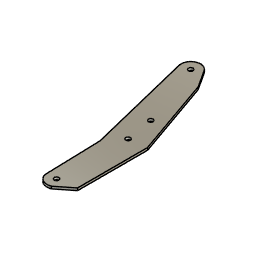
LIGHTS_SIDE_PLATE (Autodesk Fusion 360 design; units mm, degrees)
Autodesk Fusion 360 part; units mm, degrees
sketch "Esquisse1" plane through (0, 0, 0) normal (0, 0, 1) x (1, 0, 0)
  circle A0 centre (-28.9762, 57.1678) radius 4 construction
  circle A1 centre (0, 0) radius 4 construction
  circle A2 centre (65.0769, 11.2557) radius 4 construction
  spline S0 degree 3 poles (-28.9762, 70.1678) (-36.1559, 70.1678) (-41.9762, 64.3475) (-41.9762, 57.1678) (-41.9762, 49.9881) (-36.1559, 44.1678) (-28.9762, 44.1678) knots 0 0 0 0 1 1 1 2 2 2 2
  spline S1 degree 3 poles (-10.2665, 7.9748) (-2.9429, 18.3079) (-5.3826, 32.6214) (-15.7156, 39.945) (-19.5917, 42.6922) (-24.2253, 44.1678) (-28.9762, 44.1678) knots 0 0 0 0 1 1 1 2 2 2 2
  spline S2 degree 3 poles (64.1314, 172.9751) (62.374, 174.7324) (59.5248, 174.7324) (57.7674, 172.9751) (56.0101, 171.2177) (56.0101, 168.3685) (57.7674, 166.6111) knots 0 0 0 0 1 1 1 2 2 2 2
  line L0 (70.1314, 166.9751) -> (64.1314, 172.9751) construction
  spline S3 degree 3 poles (63.7674, 160.6111) (65.5248, 158.8538) (68.374, 158.8538) (70.1314, 160.6111) (71.8888, 162.3685) (71.8888, 165.2177) (70.1314, 166.9751) knots 0 0 0 0 1 1 1 2 2 2 2
  line L1 (63.7674, 160.6111) -> (57.7674, 166.6111) construction
  spline S4 degree 3 poles (48.9494, 163.7931) (48.9494, 162.9431) (49.0096, 162.0942) (49.1296, 161.2528) knots 0 0 0 0 1 1 1 1
  line L2 (57.7674, 166.6111) -> (63.7674, 160.6111) construction
  spline S5 degree 3 poles (64.1314, 172.9751) (62.374, 174.7324) (59.5248, 174.7324) (57.7674, 172.9751) (56.0101, 171.2177) (56.0101, 168.3685) (57.7674, 166.6111) knots 0 0 0 0 1 1 1 2 2 2 2 construction
  line L3 (70.1314, 166.9751) -> (64.1314, 172.9751) construction
  spline S6 degree 3 poles (63.7674, 160.6111) (65.5248, 158.8538) (68.374, 158.8538) (70.1314, 160.6111) (71.8888, 162.3685) (71.8888, 165.2177) (70.1314, 166.9751) knots 0 0 0 0 1 1 1 2 2 2 2 construction
  circle A3 centre (77.1957, 405.5301) radius 9.525 construction
  spline S7 degree 3 poles (-10.2665, 7.9748) (-2.9429, 18.3079) (-5.3826, 32.6214) (-15.7156, 39.945) (-19.5917, 42.6922) (-24.2253, 44.1678) (-28.9762, 44.1678) knots 0 0 0 0 1 1 1 2 2 2 2 construction
  spline S8 degree 3 poles (-10.2665, 7.9748) (-14.6709, 2.3048) (-13.6449, -5.8622) (-7.9748, -10.2665) (-5.0869, -12.5098) (-1.3877, -13.433) (2.2156, -12.8098) knots 0 0 0 0 1 1 1 2 2 2 2 construction
  circle A4 centre (66.9494, 163.7931) radius 4.5 construction
  circle A5 centre (66.9494, 163.7931) radius 2.95 construction
  circle A6 centre (77.1957, 405.5301) radius 6.2 construction
  arc A7 (29.3943, 70.1678) -> (38.5415, 76.1229) centre (29.3943, 80.1706) ccw construction
  circle A8 centre (105.659, 34.9839) radius 3 construction
  line L4 (30.2663, 244.3325) -> (62.716, 371.2499) construction
  line L5 (150.2746, 456.2058) -> (249.6046, 17.5293) construction
  line L6 (66.9494, 163.7931) -> (35.3654, 116.3437) construction
  circle A9 centre (86.9154, 445.0854) radius 2 construction
  line L7 (86.9154, 445.0854) -> (59.0066, 452.9658) construction
  line L8 (59.0066, 452.9658) -> (50.8545, 424.0946) construction
  line L9 (59.0066, 452.9658) -> (67.1587, 481.8369) construction
  circle A10 centre (-28.9762, 57.1678) radius 13.0029 construction
  circle A11 centre (0, 0) radius 13.0029 construction
  circle A12 centre (105.659, 34.9839) radius 13 construction
  circle A13 centre (146.3497, 66.662) radius 3 construction
  circle A14 centre (146.3497, 66.662) radius 7.5 construction
  circle A15 centre (66.9494, 163.7931) radius 13 construction
  line L10 (30.2663, 244.3325) -> (49.643, 239.3784) construction
  line L11 (49.643, 239.3784) -> (82.0927, 366.2958) construction
  line L12 (194.3502, 181.1189) -> (109.3502, 181.1189) construction
  line L13 (109.3502, 181.1189) -> (109.3502, 117.1189) construction
  line L14 (109.3502, 117.1189) -> (194.3502, 117.1189) construction
  line L15 (194.3502, 117.1189) -> (194.3502, 181.1189) construction
  line L16 (89.3502, 252.2924) -> (174.3502, 252.2924) construction
  line L17 (174.3502, 252.2924) -> (174.3502, 188.2924) construction
  line L18 (174.3502, 188.2924) -> (89.3502, 188.2924) construction
  line L19 (89.3502, 188.2924) -> (89.3502, 252.2924) construction
  arc A16 (149.7785, 59.9917) -> (116.6647, 28.0647) centre (186.2634, -10.9854) ccw construction
  arc A17 (-10.2665, 7.9748) -> (6.9982, -10.9556) centre (0, 0) ccw construction
  line L20 (115, 102) -> (155, 102) construction
  line L21 (155, 102) -> (155, 82) construction
  line L22 (155, 82) -> (115, 82) construction
  line L23 (115, 82) -> (115, 102) construction
  spline S9 degree 5 poles (47.7274, 67.4718) (47.3281, 66.25) (46.4427, 63.9241) (44.8543, 60.7877) (42.2069, 57.3229) (37.9663, 54.2531) (32.7422, 52.5151) (26.5189, 52.1302) (19.36, 53.0121) (11.3588, 55.0347) (2.6106, 58.0689) (-4.924, 61.2221) (-10.8549, 63.966) (-14.9312, 65.9611) (-17, 67) knots 0 0 0 0 0 0 0.1 0.2 0.3 0.4 0.5 0.6 0.7 0.8 0.9 1 1 1 1 1 1 construction
  arc A18 (149.7785, 59.9917) -> (145.7758, 74.1401) centre (146.3497, 66.662) ccw construction
  arc A19 (106.8583, 22.0393) -> (116.6647, 28.0647) centre (105.659, 34.9839) ccw construction
  line L24 (82.0927, 366.2958) -> (42.6573, 212.0556) construction
  spline S10 degree 5 poles (-17, 67) (-17.1898, 67.1027) (-17.5737, 67.3046) (-18.1631, 67.5968) (-18.9761, 67.9649) (-20.0408, 68.3868) (-21.1577, 68.7673) (-22.3305, 69.1037) (-23.5599, 69.3954) (-24.8424, 69.645) (-26.1736, 69.8562) (-27.2741, 69.9971) (-28.118, 70.0881) (-28.6888, 70.1423) (-28.9762, 70.1678) knots 0 0 0 0 0 0 0.1 0.2 0.3 0.4 0.5 0.6 0.7 0.8 0.9 1 1 1 1 1 1 construction
  line L25 (112.0927, 366.2958) -> (82.0927, 366.2958) construction
  circle A20 centre (0, 0) radius 4.15 construction
  circle A21 centre (-28.9762, 57.1678) radius 4.15 construction
  arc A22 (47.7274, 67.4718) -> (42.6713, 210.5165) centre (-255.8881, 128.3519) ccw construction
  circle A23 centre (66.9494, 163.7931) radius 3 construction
  circle A24 centre (110.8323, 274.6584) radius 7.5 construction
  arc A25 (106.8583, 22.0393) -> (6.9982, -10.9556) centre (128.4398, -210.8903) ccw construction
  arc A26 (82.0927, 366.2958) -> (71.4434, 397.9383) centre (52.352, 373.8997) ccw construction
  arc A27 (6.7295, -63.1083) -> (50.332, 237.2291) centre (-255.8881, 128.3519) ccw construction
  arc A28 (165.8909, 81.8045) -> (94.5564, -35.7811) centre (186.2634, -10.9854) ccw construction
  arc A29 (305.7966, -36.1174) -> (-67.5783, -57.3394) centre (128.4398, -210.8903) ccw construction
  line L26 (110.0008, 99.9968) -> (84.3502, 214.0814) construction
  arc A30 (112.5946, 267.3684) -> (84.3502, 214.0814) centre (122.0574, 228.2239) ccw construction
  arc A31 (110.0008, 99.9968) -> (145.7758, 74.1401) centre (143.1616, 108.2003) ccw construction
  line L27 (62.716, 371.2499) -> (30.2663, 244.3325) construction
  line L28 (30.2663, 244.3325) -> (-3.6429, 253.0023) construction
  line L29 (-3.6429, 253.0023) -> (28.8068, 379.9197) construction
  line L30 (28.8068, 379.9197) -> (62.716, 371.2499) construction
  line L31 (28.8068, 379.9197) -> (32.5224, 394.4522) construction
  line L32 (32.5224, 394.4522) -> (62.716, 371.2499) construction
  line L33 (-3.6429, 253.0023) -> (-7.3585, 238.4698) construction
  line L34 (-7.3585, 238.4698) -> (30.2663, 244.3325) construction
  arc A32 (112.0927, 366.2958) -> (115.0505, 280.8597) centre (180.406, 325.8915) ccw construction
  arc A33 (112.5946, 267.3684) -> (115.0505, 280.8597) centre (110.8323, 274.6584) ccw construction
  circle A34 centre (110.8323, 274.6584) radius 3 construction
  circle A35 centre (77.1957, 405.5301) radius 6 construction
  arc A36 (69.3852, 410.9818) -> (71.4434, 397.9383) centre (77.1957, 405.5301) ccw construction
  arc A37 (142.115, 85.3833) -> (84.2801, -39.8886) centre (186.2634, -10.9854) ccw construction
  arc A38 (108.2254, 142.5582) -> (166.09, 64.8957) centre (143.1616, 108.2003) ccw construction
  line L35 (69.7156, 210.791) -> (84.3502, 214.0814) construction
  line L36 (110.0008, 99.9968) -> (95.3661, 96.7063) construction
  line L37 (95.3661, 96.7063) -> (70.593, 206.8884) construction
  line L38 (65.813, 209.9136) -> (63.0859, 209.3004) construction
  line L39 (69.6598, 177.648) -> (72.9035, 178.3773) construction
  line L40 (71.751, 151.5603) -> (78.7024, 152.9702) construction
  line L41 (91.664, 95.874) -> (69.6275, 90.9193) construction
  line L42 (88.6169, 108.4898) -> (73.4183, 105.0726) construction
  line L43 (91.642, 113.2699) -> (83.4, 149.9274) construction
  line L44 (69.7156, 210.791) -> (75.9287, 183.1573) construction
  arc A39 (64.835, 180.9038) -> (60.0746, 204.4611) centre (-255.8881, 128.3519) ccw construction
  arc A40 (68.5478, 109.2108) -> (68.5529, 147.4056) centre (-255.8881, 128.3519) ccw construction
  arc A41 (58.4283, 45.7068) -> (66.5367, 87.5193) centre (-255.8881, 128.3519) ccw construction
  arc A42 (96.3504, 93.1926) -> (111.6523, 70.4686) centre (143.1616, 108.2003) ccw construction
  arc A43 (111.8948, 64.5481) -> (98.719, 48.7807) centre (186.2634, -10.9854) ccw construction
  arc A44 (95.9158, 47.0674) -> (63.299, 40.8172) centre (128.4398, -210.8903) ccw construction
  arc A45 (58.4283, 45.7068) -> (63.299, 40.8172) centre (62.2968, 44.6896) ccw construction
  arc A46 (69.6275, 90.9193) -> (66.5367, 87.5193) centre (70.505, 87.0168) ccw construction
  arc A47 (111.8948, 64.5481) -> (111.6523, 70.4686) centre (109.0884, 67.3984) ccw construction
  arc A48 (95.9158, 47.0674) -> (98.719, 48.7807) centre (95.4155, 51.036) ccw construction
  arc A49 (96.3504, 93.1926) -> (91.664, 95.874) centre (92.5414, 91.9714) ccw construction
  arc A50 (71.751, 151.5603) -> (68.5529, 147.4056) centre (72.546, 147.6401) ccw construction
  arc A51 (68.5478, 109.2108) -> (73.4183, 105.0726) centre (72.5408, 108.9752) ccw construction
  arc A52 (88.6169, 108.4898) -> (91.642, 113.2699) centre (87.7395, 112.3924) ccw construction
  arc A53 (83.4, 149.9274) -> (78.7024, 152.9702) centre (79.4974, 149.05) ccw construction
  arc A54 (72.9035, 178.3773) -> (75.9287, 183.1573) centre (72.0261, 182.2799) ccw construction
  arc A55 (64.835, 180.9038) -> (69.6598, 177.648) centre (68.7824, 181.5506) ccw construction
  arc A56 (63.0859, 209.3004) -> (60.0746, 204.4611) centre (63.9633, 205.3978) ccw construction
  arc A57 (70.593, 206.8884) -> (65.813, 209.9136) centre (66.6904, 206.011) ccw construction
  arc A58 (133.9714, 281.918) -> (103.7167, 176.372) centre (122.0574, 228.2239) ccw construction
  arc A59 (124.2253, 402.4992) -> (112.5946, 259.3587) centre (180.406, 325.8915) ccw construction
  line L45 (85.3019, 318.2923) -> (52.245, 189.4942) construction
  line L46 (78.1169, 264.0249) -> (74.6937, 264.9035) construction
  line L47 (72.533, 268.5524) -> (81.8866, 305.1363) construction
  arc A60 (87.72, 305.0513) -> (96.914, 280.5695) centre (180.406, 325.8915) ccw construction
  arc A61 (95.7143, 276.5047) -> (81.0969, 264.9286) centre (122.0574, 228.2239) ccw construction
  arc A62 (95.7143, 276.5047) -> (96.914, 280.5695) centre (94.2774, 279.1382) ccw construction
  arc A63 (87.72, 305.0513) -> (81.8866, 305.1363) centre (84.7931, 304.3932) ccw construction
  arc A64 (72.533, 268.5524) -> (74.6937, 264.9035) centre (75.4395, 267.8093) ccw construction
  arc A65 (78.1169, 264.0249) -> (81.0969, 264.9286) centre (78.8627, 266.9307) ccw construction
  arc A66 (42.6573, 212.0556) -> (42.6713, 210.5165) centre (45.5638, 211.3125) ccw construction
  circle A67 centre (86.9154, 445.0854) radius 7.5 construction
  arc A68 (94.3544, 446.0401) -> (112.0927, 366.2958) centre (365.6747, 464.5475) ccw construction
  arc A69 (69.3852, 410.9818) -> (79.4497, 445.8015) centre (7.9302, 447.6095) ccw construction
  arc A70 (94.3544, 446.0401) -> (79.4497, 445.8015) centre (86.9154, 445.0854) ccw construction
  line L48 (227.4805, 115.2371) -> (278.7067, 112.3358) construction
  line L49 (139.3502, 181.1189) -> (139.3502, 117.1189) construction
  line L50 (152.3502, 181.1189) -> (152.3502, 117.1189) construction
  line L51 (139.3502, 149.1189) -> (152.3502, 149.1189) construction
  line L52 (119.3502, 252.2924) -> (119.3502, 188.2924) construction
  line L53 (132.3502, 252.2924) -> (132.3502, 188.2924) construction
  line L54 (132.3502, 220.2924) -> (119.3502, 220.2924) construction
  circle A71 centre (110.8323, 274.6584) radius 3
  circle A72 centre (146.3497, 66.662) radius 3
  circle A73 centre (119.3502, 220.2924) radius 2.5 construction
  line L55 (155, 92) -> (147, 92) construction
  line L56 (98.4811, 272.7355) -> (132, 137)
  arc A74 (134.15, 63.9386) -> (151.2172, 55.1487) centre (146.3497, 66.662) ccw
  arc A75 (119.9733, 283.1844) -> (98.4811, 272.7355) centre (110.8323, 274.6584) ccw
  arc A76 (204.218, 109.7343) -> (203.7833, 111.288) centre (194.4019, 107.8255) ccw
  line L57 (134.15, 63.9386) -> (132, 137)
  line L58 (119.9733, 283.1844) -> (135, 260)
  line L59 (170, 70) -> (170, 160)
  line L60 (170, 160) -> (135, 260)
  line L61 (151.2172, 55.1487) -> (170, 70)
  circle A77 centre (149.3502, 129.1189) radius 2.5 construction
  circle A78 centre (141.8502, 192.2924) radius 3
  circle A79 centre (147.8502, 157.1189) radius 3
  point P0 (42.4595, 211.2822)
  point P1 (33.0466, 52.9627)
  point P2 (-22, 69)
  dimension "d3" = 5.9
  dimension "d4" = 12.4
  dimension "d49" = 6
  dimension "d53" = 131
  dimension "d64" = 4
  dimension "d68" = 29
  dimension "d69" = 30
  dimension "d70" = 30
  dimension "d71" = 26
  dimension "d72" = 6
  dimension "d73" = 15
  dimension "d74" = 26
  dimension "d75" = 20
  dimension "d76" = 30
  dimension "d77" = 160
  dimension "d78" = 64
  dimension "d79" = 85
  dimension "d80" = 64
  dimension "d81" = 85
  dimension "d82" = 20
  dimension "d83" = 40
  dimension "d86" = 8.3
  dimension "d87" = 8.3
  dimension "d88" = 6
  dimension "d89" = 15
  dimension "d93" = 79.8054
  dimension "d94" = 309.659
  dimension "d95" = 233.9273
  dimension "d97" = 325
  dimension "d98" = 95
  dimension "d99" = 249
  dimension "d104" = 35
  dimension "d105" = 15
  dimension "d106" = 15
  dimension "d107" = 6
  dimension "d108" = 12
  dimension "d109" = 106
  dimension "d111" = 49
  dimension "d112" = 15
  dimension "d113" = 4
  dimension "d114" = 4
  dimension "d115" = 4
  dimension "d116" = 4
  dimension "d117" = 4
  dimension "d118" = 55
  dimension "d119" = 95
  dimension "d121" = 3
  dimension "d122" = 3
  dimension "d123" = 3
  dimension "d124" = 3
  dimension "d131" = 3
  dimension "d132" = 15
  dimension "d133" = 74
  dimension "d135" = 55
  dimension "d137" = 42
  dimension "d138" = 42
  dimension "d139" = 13
  dimension "d141" = 5
  dimension "d142" = 8
  dimension "d153" = 35
  dimension "d154" = 55
  dimension "d156" = 5
  dimension "d157" = 10
  dimension "d158" = 20
  dimension "d164" = 6
  dimension "d165" = 22.5
  dimension "d166" = 28
  dimension "d170" = 6
  dimension "d171" = 1.5
  dimension "d172" = 28
  constraint coincident S3.start A4
  constraint coincident L0.start A4
  constraint tangent L3 A4
  constraint tangent L1 A4
  constraint concentric A4 A5
  constraint concentric A3 A6
  constraint coincident A4.centre A5.centre
  constraint coincident A9.centre L7.start
  constraint perpendicular L7 L8
  constraint perpendicular L7 L9
  constraint concentric A0 A10
  constraint concentric A8 A12
  constraint coincident A12 A19.start
  constraint concentric A13 A14
  constraint coincident A12 A16.end
  constraint concentric A4 A15
  constraint coincident L4.start L10.start
  constraint horizontal L12
  constraint vertical L13
  constraint horizontal L14
  constraint vertical L15
  constraint horizontal L16
  constraint vertical L17
  constraint horizontal L18
  constraint vertical L19
  constraint tangent A14 A16
  constraint coincident A14 A16.start
  constraint horizontal L20
  constraint vertical L21
  constraint horizontal L22
  constraint vertical L23
  constraint coincident A14 A18.end
  constraint coincident A13.centre A14.centre
  constraint coincident A8.centre A12.centre
  constraint coincident L11.end L24.start
  constraint parallel L11 L24
  constraint horizontal L25
  constraint concentric A11 A20
  constraint concentric A0 A21
  constraint coincident S9.start A22.start
  constraint concentric A4 A23
  constraint coincident A24 A30.start
  constraint tangent A12 A25
  constraint tangent L24 A26
  constraint coincident A3 A26.end
  constraint coincident A22.centre A27.centre
  constraint coincident A16.centre A28.centre
  constraint coincident A25.centre A29.centre
  constraint tangent A24 A30
  constraint tangent A14 A31
  constraint perpendicular L27 L28
  constraint parallel L27 L29
  constraint parallel L28 L30
  constraint perpendicular L10 L27
  constraint coincident L4.end L27.start
  constraint perpendicular L30 L31
  constraint perpendicular L28 L33
  constraint coincident A24 A32.end
  constraint coincident L25.start A32.start
  constraint coincident A3 A36.start
  constraint coincident A24.centre A33.centre
  constraint concentric A33 A34
  constraint concentric A3 A35
  constraint coincident A3.centre A6.centre
  constraint coincident A31.centre A38.centre
  constraint parallel L35 L36
  constraint coincident L26.end A30.end
  constraint perpendicular L26 L35
  constraint perpendicular L37 L38
  constraint perpendicular L37 L39
  constraint perpendicular L37 L41
  constraint perpendicular L37 L42
  constraint tangent A41 A45
  constraint tangent A44 A45
  constraint tangent L41 A46
  constraint tangent A41 A46
  constraint equal A45 A46
  constraint tangent A42 A47
  constraint tangent A43 A47
  constraint equal A45 A47
  constraint tangent A43 A48
  constraint tangent A44 A48
  constraint equal A45 A48
  constraint coincident L36.end L41
  constraint coincident L36.end A42
  constraint tangent A42 A49
  constraint tangent L41 A49
  constraint tangent L40 A50
  constraint tangent A40 A50
  constraint tangent L42 A51
  constraint tangent A40 A51
  constraint equal A50 A51
  constraint tangent L42 A52
  constraint tangent L43 A52
  constraint equal A50 A52
  constraint tangent L40 A53
  constraint tangent L43 A53
  constraint equal A50 A53
  constraint tangent L39 A54
  constraint tangent L44 A54
  constraint tangent L39 A55
  constraint tangent A39 A55
  constraint equal A54 A55
  constraint tangent L38 A56
  constraint tangent A39 A56
  constraint equal A54 A56
  constraint coincident L35.start L38
  constraint coincident L35.start L37
  constraint tangent L38 A57
  constraint tangent L37 A57
  constraint coincident A30.centre A58.centre
  constraint coincident A32.centre A59.centre
  constraint perpendicular L45 L46
  constraint parallel L11 L47
  constraint tangent A60 A62
  constraint tangent A61 A62
  constraint tangent L47 A63
  constraint tangent A60 A63
  constraint tangent L46 A64
  constraint tangent L47 A64
  constraint tangent L46 A65
  constraint tangent A61 A65
  constraint coincident P0 L24
  constraint coincident P0 A22
  constraint tangent L24 A66
  constraint tangent A22 A66
  constraint coincident A67 A68.start
  constraint coincident A67 A69.end
  constraint coincident L5 L48.start
  constraint coincident L12 L49.start
  constraint coincident L14 L49.end
  constraint perpendicular L14 L49
  constraint coincident L12 L50.start
  constraint coincident L14 L50.end
  constraint perpendicular L14 L50
  constraint midpoint L49 L51.start
  constraint midpoint L50 L51.end
  constraint coincident L16 L52.start
  constraint coincident L18 L52.end
  constraint perpendicular L18 L52
  constraint coincident L16 L53.start
  constraint coincident L18 L53.end
  constraint perpendicular L18 L53
  constraint midpoint L53 L54.start
  constraint midpoint L52 L54.end
  constraint concentric A34 A71
  constraint concentric A14 A72
  constraint coincident L54.end A73.centre
  constraint midpoint L21 L55.start
  constraint perpendicular L21 L55
  constraint coincident A58 A75.start
  measures "d3" diameter of A5
  measures "d4" diameter of A6
  measures "d49" diameter of A8
  measures "d53" distance of L4.start L4.end
  measures "d64" diameter of A9
  measures "d68" distance of A9.centre L7.end
  measures "d69" distance of L7.end L8.end
  measures "d70" distance of L7.end L9.end
  measures "d71" diameter of A12
  measures "d72" diameter of A13
  measures "d73" diameter of A14
  measures "d74" diameter of A15
  measures "d75" distance of L4.end L11.end
  measures "d76" distance of L11.end L25.start
  measures "d77" distance of L11.end P0
  measures "d78" distance of L12.start L14.end
  measures "d79" distance of L12.start L12.end
  measures "d80" distance of L16.start L18.end
  measures "d81" distance of L16.start L16.end
  measures "d82" distance of L20.start L22.end
  measures "d83" distance of L20.start L20.end
  measures "d86" diameter of A20
  measures "d87" diameter of A21
  measures "d88" diameter of A23
  measures "d89" diameter of A24
  measures "d93" radius of A16
  measures "d94" radius of A22
  measures "d95" radius of A25
  measures "d97" radius of A27
  measures "d98" radius of A28
  measures "d99" radius of A29
  measures "d104" distance of L4.end L29.end
  measures "d105" distance of L29.end L31.end
  measures "d106" distance of L28.end L33.end
  measures "d107" diameter of A34
  measures "d108" diameter of A35
  measures "d109" radius of A37
  measures "d111" radius of A38
  measures "d112" distance of L26.end L35.start
  measures "d113" radius of A45
  measures "d114" radius of A49
  measures "d115" radius of A50
  measures "d116" radius of A54
  measures "d117" radius of A57
  measures "d118" radius of A58
  measures "d119" radius of A59
  measures "d121" radius of A62
  measures "d122" radius of A63
  measures "d123" radius of A64
  measures "d124" radius of A65
  measures "d131" radius of A66
  measures "d132" diameter of A67
  measures "d133" angle of L5 L48
  measures "d135" distance of L15 L49
  measures "d137" distance of L15 L50
  measures "d138" distance of L17 L53
  measures "d139" distance of L52 L53
  measures "d141" diameter of A73
  measures "d142" distance of L55.start L55.end
  measures "d153" horizontal distance of L26.end L54.end
  measures "d154" horizontal distance of L26.end L51.start
  measures "d156" diameter of A77
  measures "d157" horizontal distance of L51.start A77.centre
  measures "d158" vertical distance of L51.start A77.centre
  measures "d164" diameter of A78
  measures "d165" horizontal distance of L54.end A78.centre
  measures "d166" vertical distance of L54.end A78.centre
  measures "d170" diameter of A79
  measures "d171" horizontal distance of A77.centre A79.centre
  measures "d172" vertical distance of A77.centre A79.centre
extrude "Extrusion2" add sketch "Esquisse1" along normal blind 3
equation "d135 = 42 mm + 13 mm"
